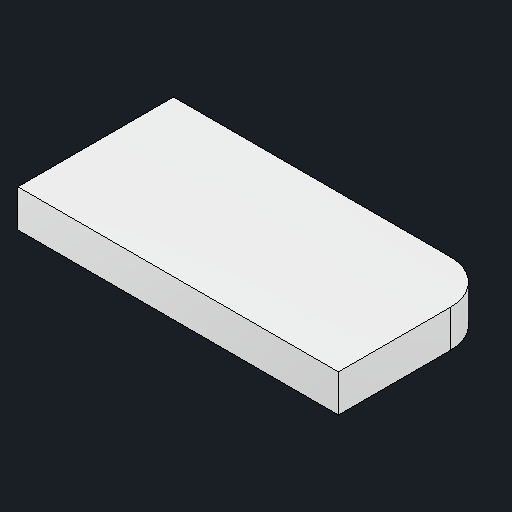
# Autodesk Inventor part: Przegroda
Saved by Autodesk Inventor 2023 (Build 270158000, 158)
## iProperties
Created: 2024-02-25
Part Number: Przegroda
Material: Aluminum 6061
Document SubType Name: Modeling
Designer: Michał
Density: 2.7 g/cm^3
Appearance: Aluminum - Flat
Author: Michał
Autodesk Inventor part; units mm, degrees
ref_plane "YZ Plane" through (0, 0, 0) normal (1, 0, 0) x (0, 1, 0)
ref_plane "XZ Plane" through (0, 0, 0) normal (0, 1, 0) x (-1, 0, 0)
ref_plane "XY Plane" through (0, 0, 0) normal (0, 0, 1) x (1, 0, 0)
sketch "Sketch1" plane through (0, 0, 0) normal (0, 0, 1) x (1, 0, 0)
  line L0 (-18.5543, 18.8307) -> (32.9457, 18.8307)
  line L1 (32.9457, 18.8307) -> (32.9457, 12.8307)
  line L2 (32.9457, 12.8307) -> (-18.5543, 12.8307)
  line L3 (-18.5543, 12.8307) -> (-18.5543, 18.8307)
  line L4 (-64.2543, 64.8307) -> (-64.2543, -33.1693) construction
  line L5 (32.9457, 15.8307) -> (-64.2543, 15.8307) construction
  line L6 (9.4457, -32.9193) -> (9.4457, 64.5807) construction
  point P0 (32.9457, 15.8307)
  dimension "d2" = 51.5
  dimension "d3" = 6
  dimension "d4" = 23.5
  constraints: 10 end point, 2 midpoint, 2 parallel, 1 coincident, 1 horizontal, 1 perpendicular, 1 other
  measures "d2" distance from line of point (32.946, 15.831) L3
  measures "d3" distance between parallel lines of L2 L0
  measures "d4" distance between parallel lines of L1 L6
extrude "Extrusion1" add sketch "Sketch1" along normal blind 25
sketch "Sketch2" plane through (0, 0, 0) normal (0, 0, -1) x (-1, 0, 0)
  line L0 (18.5543, 18.8307) -> (18.5543, 12.8307) construction
  point P0 (0, 0)
  point P1 (-1.4457, 15.8307)
  point P2 (18.5543, 15.8307)
  dimension "d5" = 20
  constraints: 1 horizontal alignment, 1 midpoint
  measures "d5" distance from line of L0 point (-1.446, 15.831)
hole "Hole1" at (1.4457, 15.8307, 0) direction (0, 0, 1) diameter 2.459 depth 6 tip angle 118 thread size "M3x0.5" class "6H" standard "ISO Metric profile"
extrude "Extrusion2" [suppressed]
fillet "Fillet1" radius 7 1 edges at (32.9457, 15.8307, 0)
body "Solid1"
